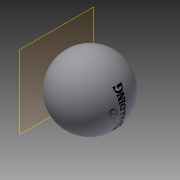
# Autodesk Inventor part: soccer ball
Saved by Autodesk Inventor 2015 (Build 190159000, 159)
## iProperties
Created: 2015-09-25
Part Number: soccer ball
Material: Generic
Document SubType Name: Modeling
Designer: Brian
Appearance: Default
Surface Area: 1520.53 cm^2
Volume: 5575.28 cm^3
Author: Brian
Autodesk Inventor part; units mm, degrees
ref_plane "XZ Plane" through (0, 0, 0) normal (0, 1, 0) x (-1, 0, 0)
ref_plane "XY Plane" through (0, 0, 0) normal (0, 0, 1) x (1, 0, 0)
sketch "Sketch1" plane through (0, 0, 0) normal (0, 1, 0) x (-1, 0, 0)
  circle A0 centre (0, 0) radius 110 construction
  line L0 (0, 110) -> (0, -110)
  arc A1 (0, -110) -> (0, 110) centre (0, 0) ccw
  dimension "d0" = 220
  constraints: 4 point on circle, 2 centre point, 2 coincident, 2 end point, 1 midpoint, 1 vertical
  measures "d0" diameter of A0
revolve "Revolution1" add sketch "Sketch1" angle 360 about axis through (0, 0, 110) along (0, 0, -1)
ref_plane "Work Plane1" through (-110, 0, 0) normal (1, 0, 0) x (0, 1, 0)
sketch "Sketch2" plane through (-110, 0, 0) normal (1, 0, 0) x (0, 1, 0)
  line L0 (-42.6714, -69.5221) -> (-42.6714, 68.6646) construction
  line L1 (-42.6714, 68.6646) -> (18.4762, 68.6646) construction
  line L2 (18.4762, 68.6646) -> (18.4762, -69.5221) construction
  line L3 (18.4762, -69.5221) -> (-42.6714, -69.5221) construction
  point P0 (0, 0)
  constraints: 2 other
decal "Decal1"
body "Solid1"
